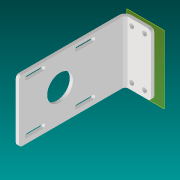
# Autodesk Inventor part: steppermount
Saved by Autodesk Inventor 2020.3 (Build 243373000, 373)
## iProperties
Created: 2020-05-24
Part Number: steppermount
Material: Generic
Document SubType Name: Sheet Metal
Designer: Svend
Mass: 5.66404 g
Surface Area: 65.4079 cm^2
Volume: 5.66404 cm^3
Density: 1 g/cm^3
Sheet Metal Rule: Default_mm
Appearance: Default
Author: Svend
Autodesk Inventor part; units mm, degrees
ref_plane "YZ Plane" through (0, 0, 0) normal (1, 0, 0) x (0, 1, 0)
ref_plane "XZ Plane" through (0, 0, 0) normal (0, 1, 0) x (-1, 0, 0)
ref_plane "XY Plane" through (0, 0, 0) normal (0, 0, 1) x (1, 0, 0)
ref_plane "Work Plane1" through (0, 0, 0) normal (0, 0, 1) x (1, 0, 0)
sketch "Sketch1" plane through (0, 0, 0) normal (0, 0, 1) x (1, 0, 0)
  circle A0 centre (-8, -36) radius 1.5
  circle A1 centre (-8, -6) radius 1.5
  circle A2 centre (-15.9281, -36) radius 1.5
  circle A3 centre (-15.9281, -6) radius 1.5
  line L0 (-19.9281, -2) -> (1.2168, -2)
  line L1 (-19.9281, -40) -> (-19.9281, -2)
  line L2 (-0.2416, -40) -> (-19.9281, -40)
  line L3 (-0.2416, -40) -> (-0.2416, -30)
  line L4 (-0.2416, -30) -> (0, -30)
  line L5 (0, -5) -> (0, -30)
  spline S0 degree 3 poles (1.2168, -2) (1.1498, -2.0729) (1.0846, -2.1482) (0.788, -2.5121) (0.5885, -2.8262) (0.3051, -3.4054) (0.1887, -3.7185) (0.036, -4.3634) (0, -4.6952) (0, -5) knots 0 0 0 0 0.087816 0.087816 0.414412 0.414412 0.707206 0.707206 1 1 1 1
  line L6 (-19.9281, -2) -> (-3.9281, -2)
  line L7 (-3.9281, -2) -> (-3.9281, -40)
  line L8 (-3.9281, -40) -> (-19.9281, -40)
  line L9 (-19.9281, -40) -> (-19.9281, -2)
  point P0 (0, 0)
  dimension "d0" = 16
  measures "d0" distance between parallel lines of L1 L7
extrude "Plate1" add sketch "Sketch1" along normal blind 2 contours L0 L7 L2 L1
sketch "Sketch2" plane through (-19.9281, -40, 2) normal (-1, 0, 0) x (0, -1, 0)
  line L0 (-38, 0) -> (0, 0)
  line L1 (0, 0) -> (0, 66)
  line L2 (0, 66) -> (-38, 66)
  line L3 (-38, 66) -> (-38, 0)
  constraints: 6 end point, 1 horizontal, 1 perpendicular, 1 vertical
edge flange "Flange1" height 68 angle 90 thickness 2 bend radius 2 thickness toward (-1, 0, 0) relief straight relief width 2 relief depth 1 edges at (-19.9281, -21, 2) wall of the first edge with corners at (-19.9281, -2, 2) (-19.9281, -40, 2) (-19.9281, -40, 68) (-19.9281, -2, 68)
bend "Bend1"
corner "Corner1"
sketch "Sketch3" plane through (-21.9281, -40, 68) normal (-1, 0, 0) x (0, 0, 1)
  circle A0 centre (-10.0213, 3.75) radius 1.25 projected
  circle A1 centre (-41.0213, 3.75) radius 1.25 projected
  circle A2 centre (-41.0213, 34.75) radius 1.25 projected
  circle A3 centre (-10.0213, 34.75) radius 1.25 projected
  circle A4 centre (-25.5213, 19.25) radius 6 projected
  line L0 (-46.0213, 3.75) -> (-36.0213, 3.75) construction
  line L1 (-46.0213, 2.5) -> (-36.0213, 2.5)
  line L2 (-36.0213, 5) -> (-46.0213, 5)
  arc A5 (-46.0213, 5) -> (-46.0213, 2.5) centre (-46.0213, 3.75) ccw
  arc A6 (-36.0213, 2.5) -> (-36.0213, 5) centre (-36.0213, 3.75) ccw
  line L3 (-46.0213, 34.75) -> (-36.0213, 34.75) construction
  line L4 (-46.0213, 33.5) -> (-36.0213, 33.5)
  line L5 (-36.0213, 36) -> (-46.0213, 36)
  arc A7 (-46.0213, 36) -> (-46.0213, 33.5) centre (-46.0213, 34.75) ccw
  arc A8 (-36.0213, 33.5) -> (-36.0213, 36) centre (-36.0213, 34.75) ccw
  line L6 (-15.0213, 34.75) -> (-5.0213, 34.75) construction
  line L7 (-15.0213, 33.5) -> (-5.0213, 33.5)
  line L8 (-5.0213, 36) -> (-15.0213, 36)
  arc A9 (-15.0213, 36) -> (-15.0213, 33.5) centre (-15.0213, 34.75) ccw
  arc A10 (-5.0213, 33.5) -> (-5.0213, 36) centre (-5.0213, 34.75) ccw
  line L9 (-15.0213, 3.75) -> (-5.0213, 3.75) construction
  line L10 (-15.0213, 2.5) -> (-5.0213, 2.5)
  line L11 (-5.0213, 5) -> (-15.0213, 5)
  arc A11 (-15.0213, 5) -> (-15.0213, 2.5) centre (-15.0213, 3.75) ccw
  arc A12 (-5.0213, 2.5) -> (-5.0213, 5) centre (-5.0213, 3.75) ccw
  circle A13 centre (-25.5213, 19.25) radius 8
  point P0 (-68, 40)
  dimension "d12" = 5
  dimension "d13" = 5
  dimension "d14" = 5
  dimension "d15" = 5
  dimension "d16" = 16
  constraints: 32 end point, 20 tangent, 16 point on circle, 9 centre point, 5 parallel, 4 midpoint, 2 point on line, 1 coincident, 1 horizontal
  measures "d12" distance of A1.centre L0.end
  measures "d13" distance of A2.centre L3.end
  measures "d14" distance of A3.centre L6.end
  measures "d15" distance of A0.centre L9.end
  measures "d16" diameter of A13
extrude "Cut1" cut sketch "Sketch3" against normal blind 2 contours A0 | A0 L11 A12 L10 | A0 L10 A11 L11 | A1 | A1 L2 A6 L1 | A1 L1 A5 L2 | A2 | A2 L5 A8 L4 | A2 L4 A7 L5 | A3 | A3 L8 A10 L7 | A3 L7 A9 L8 | A4 | A13
fillet "Corner Round1" radius 2 4 edges at (-20.9281, -40, 68) (-20.9281, -2, 68) (-3.9281, -2, 1) (-3.9281, -40, 1)
equation "\"d17\" = Thickness"
equation "\"d1\" = Thickness"
equation "\"d2\" = BendReliefWidth"
equation "\"d3\" = BendReliefDepth"
equation "\"d4\" = MinimumRemnant"
equation "\"d5\" = TransitionRadius"
equation "\"d8\" = BendRadius"
equation "\"d9\" = CornerReliefSize"
equation "\"d10\" = GapSize"
equation "\"d11\" = JacobiRadiusSize"
equation "\"BendRadius\" = Thickness"
equation "\"BendReliefWidth\" = Thickness"
equation "\"BendReliefDepth\" = 0.5 * Thickness"
equation "\"CornerReliefSize\" = 4 * Thickness"
equation "\"MinimumRemnant\" = 2 * Thickness"
equation "\"TransitionRadius\" = BendRadius"
equation "\"JacobiRadiusSize\" = BendRadius"
equation "\"GapSize\" = Thickness"
equation "\"Thickness\" = 2"
body "Solid1"
